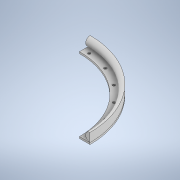
# Autodesk Inventor part: Whack01-RunnerForFrisbeeShooter
Saved by Autodesk Inventor 2022 (Build 260153000, 153)
## iProperties
Created: 2021-04-23
Part Number: Whack01-RunnerForFrisbeeShooter
Material: Generic
Document SubType Name: Modeling
Designer: robst
Density: 1 g/cm^3
Appearance: Default
Author: robst
Autodesk Inventor part; units mm, degrees
ref_plane "YZ Plane" through (0, 0, 0) normal (1, 0, 0) x (0, 1, 0)
ref_plane "XZ Plane" through (0, 0, 0) normal (0, 1, 0) x (-1, 0, 0)
ref_plane "XY Plane" through (0, 0, 0) normal (0, 0, 1) x (1, 0, 0)
sketch "Sketch2" plane through (0, 0, 0) normal (0, 0, 1) x (1, 0, 0)
  line L0 (304.8, 0) -> (304.8, 31.75)
  arc A0 (304.8, 31.75) -> (304.8, 0) centre (304.8, 15.875) ccw
  line L1 (304.8, 0) -> (266.7, 0)
  line L2 (266.7, 0) -> (266.7, -6.35)
  line L3 (266.7, -6.35) -> (304.8, -6.35)
  line L4 (304.8, -6.35) -> (304.8, 0)
  line L5 (0, 0) -> (304.8, 0) construction
  line L6 (0, -13.97) -> (0, 39.37) projected
  dimension "d0" = 31.75
  dimension "d1" = 304.8
  dimension "d2" = 6.35
  dimension "d8" = 15.875
  dimension "d9" = 38.1
  constraints: 12 end point, 4 perpendicular, 2 point on circle, 1 centre point, 1 collinear, 1 horizontal, 1 point on line, 1 vertical
  measures "d0" distance of L0.start L0.end
  measures "d1" distance from line of L5.start L0
  measures "d2" distance of L3.end L0.start
  measures "d8" radius of A0
  measures "d9" distance between parallel lines of L2 L4
revolve "Revolution1" add sketch "Sketch2" angle 90 about axis through (0, -10, 0) along (0, 1, 0)
sketch "Sketch4" plane through (266.7, 0, 0) normal (0, 1, 0) x (1, 0, 0)
  line L0 (38.1, 0) -> (0, 0) projected
  point P0 (-266.7, 0)
  point P1 (11.5431, 25.4)
  dimension "d10" = 279.4
  dimension "d18" = 25.4
  measures "d10" distance of point (11.543, 25.4) point (-266.7, 0)
  measures "d18" distance from line of point (11.543, 25.4) L0
hole "Hole1" at (278.2431, 0, -25.4) direction (0, -1, 0) diameter 5.6134 end through all counterbore diameter 9.525 counterbore depth 3.048 clearance for "Hex Machine Screw" size "#10" standard "Ansi Unified Screw Threads"
pattern_circular "Circular Pattern1" count 6 over 80 about axis through (0, -10, 0) along (0, 1, 0) of "Hole1"
sketch "Sketch3" plane through (0, -6.35, -266.7) normal (-1, 0, 0) x (0, 0, 1)
  arc A0 (-38.1, 6.35) -> (-38.1, 38.1) centre (-38.1, 22.225) ccw projected
  line L0 (-38.1, 38.1) -> (-38.1, 6.35) projected
  line L1 (-38.1, 6.35) -> (-38.1, 38.1)
  line L2 (-38.1, 0) -> (0, 0) projected
  line L3 (-38.1, 6.35) -> (-38.1, 0)
  line L4 (-38.1, 0) -> (0, 0)
  line L5 (0, 6.35) -> (-38.1, 6.35)
  arc A1 (-38.1, 6.35) -> (-38.1, 38.1) centre (-38.1, 22.225) ccw
  line L6 (266.7, 6.35) -> (0, 6.35) projected
  line L7 (0, 0) -> (0, 6.35) projected
  line L8 (0, 6.35) -> (0, 0)
  constraints: 10 end point, 3 equal length, 2 point on circle, 2 vertical, 1 centre point, 1 concentric
equation "\"d1\" = outerRadius"
equation "\"d8\" = spacerRadius"
equation "\"wheelDiameter\" = 184.15"
equation "\"frisbeeDiameter\" = 228.6"
equation "\"outerRadius\" = 304.8"
equation "\"wheelRadius\" = 0.5 * wheelDiameter"
equation "\"spacerRadius\" = 15.875"
body "Solid1"
